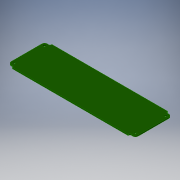
# Autodesk Inventor part: MainPCB
Saved by Autodesk Inventor 2017 (Build 210142000, 142)
## iProperties
Created: 2017-04-14
Part Number: MainPCB
Material: Generic
Document SubType Name: Sheet Metal
Designer: jeffkub
Density: 1 g/cm^3
Sheet Metal Rule: Default_mm
Appearance: Default(2)
Author: jeffkub
Autodesk Inventor part; units mm, degrees
ref_plane "YZ Plane" through (0, 0, 0) normal (1, 0, 0) x (0, 1, 0)
ref_plane "XZ Plane" through (0, 0, 0) normal (0, 1, 0) x (-1, 0, 0)
ref_plane "XY Plane" through (0, 0, 0) normal (0, 0, 1) x (1, 0, 0)
sketch "Sketch2" plane through (0, 0, 0) normal (0, 1, 0) x (-1, 0, 0)
  line L0 (101.6465, 0) -> (-102.4493, 0)
  line L1 (0, -49.7697) -> (0, 40.9396)
  line L2 (0, -27.5) -> (80, -27.5)
  line L3 (88, -27.5) -> (88, -25) construction
  line L4 (84, -25) -> (82, -25)
  line L5 (80.5, -26.5) -> (80.5, -27)
  line L6 (88, -21) -> (88, 0)
  line L7 (80.5, -27.5) -> (88, -27.5) construction
  arc A0 (84, -25) -> (88, -21) centre (84, -21) ccw
  arc A1 (82, -25) -> (80.5, -26.5) centre (82, -26.5) ccw
  arc A2 (80, -27.5) -> (80.5, -27) centre (80, -27) ccw
  circle A3 centre (84, -21) radius 1.6
  point P0 (0, 0)
  dimension "d7" = 176
  dimension "d8" = 55
  dimension "d9" = 2.5
  dimension "d10" = 7.5
  dimension "d11" = 4
  dimension "d12" = 1.5
  dimension "d13" = 0.5
  dimension "d16" = 3.2
  constraints: 16 end point, 8 point on line, 6 point on circle, 6 tangent, 4 centre point, 4 horizontal, 4 perpendicular, 1 coincident, 1 vertical
  measures "d7" diameter of L3 L1
  measures "d8" diameter of L2 L0
  measures "d9" distance between parallel lines of L4 L2
  measures "d10" distance between parallel lines of L5 L3
  measures "d11" radius of A0
  measures "d12" radius of A1
  measures "d13" radius of A2
  measures "d16" diameter of A3
extrude "Extrusion1" add sketch "Sketch2" along normal blind 1.6
mirror "Mirror1" about plane through (0, 0, 0) normal (0, 0, 1) of "Extrusion1"
mirror "Mirror2" about plane through (0, 0, 0) normal (1, 0, 0) of "Extrusion1", "Mirror1"
equation "\"BendRadius\" = Thickness"
equation "\"BendReliefWidth\" = Thickness"
equation "\"BendReliefDepth\" = 0.5 * Thickness"
equation "\"CornerReliefSize\" = 4 * Thickness"
equation "\"MinimumRemnant\" = 2 * Thickness"
equation "\"TransitionRadius\" = BendRadius"
equation "\"JacobiRadiusSize\" = BendRadius"
equation "\"GapSize\" = Thickness"
equation "\"Thickness\" = 0.5"
body "Solid1"
